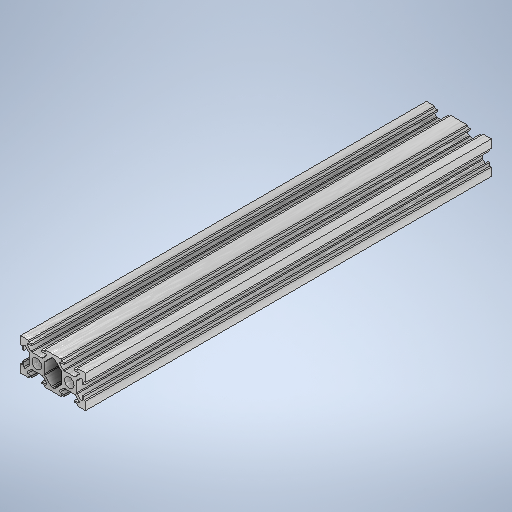
# Autodesk Inventor part: 20x40mm_perfil
Saved by Autodesk Inventor 2025.2 (Build 292293000, 293)
## iProperties
Created: 2025-04-10
Part Number: 20x40mm_perfil
Material: Aço
Document SubType Name: Modeling
Designer: Formação
Density: 7.85 g/cm^3
Appearance: Polido escovado
Author: Formação
Autodesk Inventor part; units mm, degrees
ref_plane "YZ Plane" through (0, 0, 0) normal (1, 0, 0) x (0, 1, 0)
ref_plane "XZ Plane" through (0, 0, 0) normal (0, 1, 0) x (-1, 0, 0)
ref_plane "XY Plane" through (0, 0, 0) normal (0, 0, 1) x (1, 0, 0)
sketch "Esboço1" plane through (0, 0, 0) normal (0, 0, 1) x (1, 0, 0)
  line L0 (1376.0742, -3.2) -> (1376.0729, -2.2)
  line L1 (-14.9742, 1386.056) -> (-13.9742, 1386.056)
  line L2 (-13.9742, 1386.056) -> (-13.9742, 1387.2256)
  line L3 (-13.9742, 1387.2256) -> (-15.9742, 1387.2256)
  line L4 (1376.0625, 5) -> (1376.0625, 4)
  line L5 (1376.0625, 4) -> (2769.8011, 4)
  line L6 (2769.8011, 4) -> (2769.8055, 6)
  arc A0 (-16.3152, 1388.0487) -> (-15.9742, 1387.2256) centre (-15.9742, 1387.7078) ccw
  line L7 (-14.9742, -1386.056) -> (-13.9742, -1386.056)
  line L8 (-13.9742, -1386.056) -> (6.3334, -2779.6467)
  line L9 (6.3334, -2779.6467) -> (4.3336, -2779.6758)
  arc A1 (4.3336, -2779.6758) -> (4.0107, -2780.3971) centre (4.3399, -2780.1116) ccw
  line L10 (4.0107, -2780.3971) -> (5.4731, -2781.7335)
  arc A2 (2770.6738, 6.0529) -> (2769.8055, 6) centre (2770.2413, 5.999) ccw
  line L11 (-20, 10) -> (0, 10) construction
  line L12 (0, 10) -> (0, -10) construction
  line L13 (0, -10) -> (-20, -10) construction
  line L14 (-20, -10) -> (-20, 10) construction
  line L15 (-20, 10) -> (0, -10) construction
  line L16 (0, 10) -> (-20, -10) construction
  line L17 (0, 10) -> (20, 10) construction
  line L18 (20, 10) -> (20, -10) construction
  line L19 (20, -10) -> (0, -10) construction
  line L20 (0, -10) -> (0, 10) construction
  line L21 (0, 10) -> (20, -10) construction
  line L22 (20, 10) -> (0, -10) construction
  circle A3 centre (-10, 0) radius 3 construction
  circle A4 centre (10, 0) radius 3 construction
  line L23 (-20, 10) -> (-20, 5)
  line L24 (-20, -10) -> (-20, -5)
  line L25 (-20, -5) -> (-19, -5)
  line L26 (-19, -5) -> (-19, -3.1)
  line L27 (-19, -3.1) -> (-18, -3.1)
  line L28 (-20, 5) -> (-19, 5)
  line L29 (-19, 5) -> (-19, 3.1)
  line L30 (-19, 3.1) -> (-18, 3.1)
  line L31 (20, -10) -> (20, -5)
  line L32 (20, -5) -> (19, -5)
  line L33 (19, -5) -> (19, -3.1)
  line L34 (19, -3.1) -> (18, -3.1)
  line L35 (20, 10) -> (20, 5)
  line L36 (20, 5) -> (19, 5)
  line L37 (19, 5) -> (19, 3.1)
  line L38 (19, 3.1) -> (18, 3.1)
  line L39 (-18, 3.1) -> (-18, 5.6)
  line L40 (-18, -3.1) -> (-18, -5.6)
  line L41 (18, -3.1) -> (18, -5.6)
  line L42 (18, 3.1) -> (18, 5.6)
  arc A5 (18, 5.6) -> (17.0646, 5.9536) centre (17.4655, 5.6) ccw
  line L43 (-20, -10) -> (-15, -10)
  line L44 (-20, 10) -> (-15, 10)
  line L45 (-15, 10) -> (-15, 9)
  line L46 (-15, 9) -> (-13.1, 9)
  line L47 (-13.1, 9) -> (-13.1, 8)
  line L48 (-13.1, 8) -> (-15.6, 8)
  line L49 (-15, -10) -> (-15, -9)
  line L50 (-15, -9) -> (-13.1, -9)
  line L51 (-13.1, -9) -> (-13.1, -8)
  line L52 (-13.1, -8) -> (-15.6, -8)
  line L53 (-20, 0) -> (20, 0) construction
  line L54 (20, -10) -> (15, -10)
  line L55 (15, -10) -> (15, -9)
  line L56 (15, -9) -> (13.1, -9)
  line L57 (13.1, -9) -> (13.1, -8)
  line L58 (13.1, -8) -> (15.6, -8)
  line L59 (20, 10) -> (15, 10)
  arc A6 (-17.1464, 5.9536) -> (-18, 5.6) centre (-17.5, 5.6) ccw
  arc A7 (-15.9536, -7.1464) -> (-15.6, -8) centre (-15.6, -7.5) ccw
  arc A8 (15.6, -8) -> (15.9536, -7.1464) centre (15.6, -7.5) ccw
  arc A9 (-13.1, -4.6243) -> (-13.6657, -4.8586) centre (-13.1, -5.4243) ccw
  line L60 (-15.9536, -7.1464) -> (-13.6657, -4.8586)
  arc A10 (-18, -5.6) -> (-17.1465, -5.9536) centre (-17.5, -5.6) ccw
  line L61 (-14.6243, 3.1) -> (-14.6243, -3.1) construction
  arc A11 (-14.8586, -3.6657) -> (-14.6243, -3.1) centre (-15.4243, -3.1) ccw
  line L62 (-17.1465, -5.9536) -> (-14.8586, -3.6657)
  arc A12 (-15.6, 8) -> (-15.9536, 7.1464) centre (-15.6, 7.5) ccw
  line L63 (-14.6243, 3.1) -> (-14.6243, -3.1)
  arc A13 (-14.6243, 3.1) -> (-14.8586, 3.6657) centre (-15.4243, 3.1) ccw
  line L64 (-17.1464, 5.9536) -> (-14.8586, 3.6657)
  line L65 (-14.8586, 3.6657) -> (-14.8586, 3.6657)
  arc A14 (-13.6657, 4.8586) -> (-13.1, 4.6243) centre (-13.1, 5.4243) ccw
  line L66 (-15.9536, 7.1464) -> (-13.6657, 4.8586)
  line L67 (-6.9, -9) -> (-6.9, -8)
  line L68 (-6.9, -8) -> (-4.4, -8)
  line L69 (-6.9, -9) -> (-5, -9)
  line L70 (-5, -9) -> (-5, -10)
  line L71 (-10, 0) -> (-10, -10) construction
  arc A15 (-4.4, -8) -> (-4.0464, -7.1464) centre (-4.4, -7.5) ccw
  line L72 (-4.0464, -7.1464) -> (-6.3343, -4.8586)
  arc A16 (-6.3343, -4.8586) -> (-6.9, -4.6243) centre (-6.9, -5.4243) ccw
  line L73 (-13.1, -4.6243) -> (-6.9, -4.6243)
  line L74 (-13.1, 4.6243) -> (-6.9, 4.6243)
  arc A17 (-6.9, 4.6243) -> (-6.3343, 4.8586) centre (-6.9, 5.4243) ccw
  line L75 (-6.3343, 4.8586) -> (-4.0464, 7.1464)
  arc A18 (-4.0464, 7.1464) -> (-4.4, 8) centre (-4.4, 7.5) ccw
  line L76 (-4.4, 8) -> (-6.9, 8)
  line L77 (-6.9, 8) -> (-6.9, 9)
  line L78 (-6.9, 9) -> (-5, 9)
  line L79 (-5, 9) -> (-5, 10)
  line L80 (15, 10) -> (15, 9)
  line L81 (15, 9) -> (13.1, 9)
  line L82 (13.1, 9) -> (13.1, 8)
  line L83 (13.1, 8) -> (15.6, 8)
  arc A19 (15.9536, 7.1464) -> (15.6, 8) centre (15.6, 7.5) ccw
  arc A20 (17.1464, -5.9536) -> (18, -5.6) centre (17.5, -5.6) ccw
  line L84 (13.6657, -4.8586) -> (15.9536, -7.1464)
  line L85 (17.1464, -5.9536) -> (14.8586, -3.6657)
  arc A21 (14.6247, -3.0725) -> (14.8586, -3.6657) centre (15.4243, -3.1) ccw
  arc A22 (13.6657, -4.8586) -> (13.1, -4.6243) centre (13.1, -5.4243) ccw
  line L86 (15.9536, 7.1464) -> (13.6657, 4.8586)
  arc A23 (13.1, 4.6243) -> (13.6657, 4.8586) centre (13.1, 5.4243) ccw
  line L87 (17.0646, 5.9536) -> (14.7767, 3.6657)
  arc A24 (14.7767, 3.6657) -> (14.6247, 3.0725) centre (15.4167, 3.1857) ccw
  line L88 (14.6247, 3.0725) -> (14.6247, -3.0725)
  line L89 (13.1, -4.6243) -> (6.8983, -4.6243)
  arc A25 (6.8983, -4.6243) -> (6.3326, -4.8586) centre (6.8983, -5.4243) ccw
  line L90 (6.3326, -4.8586) -> (4.0448, -7.1464)
  arc A26 (4.0448, -7.1464) -> (4.3983, -8) centre (4.3983, -7.5) ccw
  line L91 (13.1, 4.6243) -> (6.8983, 4.6243)
  arc A27 (6.3326, 4.8586) -> (6.8983, 4.6243) centre (6.8983, 5.4243) ccw
  line L92 (6.3326, 4.8586) -> (4.0448, 7.1464)
  arc A28 (4.3983, 8) -> (4.0448, 7.1464) centre (4.3983, 7.5) ccw
  line L93 (4.3983, 8) -> (6.8983, 8)
  line L94 (4.3983, -8) -> (6.8983, -8)
  line L95 (6.8983, 8) -> (6.8983, 9)
  line L96 (6.8983, 9) -> (4.9983, 9)
  line L97 (4.9983, 9) -> (4.9983, 10)
  line L98 (-5, 10) -> (4.9983, 10)
  line L99 (6.8983, -8) -> (6.8983, -9)
  line L100 (6.8983, -9) -> (5, -9)
  line L101 (5, -9) -> (5, -10)
  line L102 (-5, -10) -> (5, -10)
  line L103 (-5.3777, 3.1) -> (-5.3777, -3.1)
  arc A29 (-5.1434, 3.6657) -> (-5.3777, 3.1) centre (-4.5777, 3.1) ccw
  line L104 (-5.1434, 3.6657) -> (-1.1176, 7.6913)
  arc A30 (-0.3722, 8) -> (-1.1176, 7.6913) centre (-0.3723, 6.9459) ccw
  line L105 (-0.3722, 8) -> (0.3723, 8)
  arc A31 (-5.3777, -3.1) -> (-5.1434, -3.6657) centre (-4.5777, -3.1) ccw
  line L106 (-5.1434, -3.6657) -> (-1.1176, -7.6913)
  arc A32 (-1.1176, -7.6913) -> (-0.3723, -8) centre (-0.3723, -6.9459) ccw
  line L107 (-0.3723, -8) -> (0.3723, -8)
  arc A33 (0.3723, -8) -> (1.1176, -7.6913) centre (0.3723, -6.9459) ccw
  line L108 (1.1176, -7.6913) -> (5.1434, -3.6657)
  arc A34 (5.1434, -3.6657) -> (5.3777, -3.1) centre (4.5777, -3.1) ccw
  line L109 (5.3777, -3.1) -> (5.3777, 3.1)
  arc A35 (5.3777, 3.1) -> (5.1435, 3.6656) centre (4.5777, 3.1) ccw
  line L110 (5.1435, 3.6656) -> (1.1178, 7.6913)
  arc A36 (1.1178, 7.6913) -> (0.3723, 8) centre (0.3725, 6.946) ccw
  circle A37 centre (-10, 0) radius 3
  circle A38 centre (10, 0) radius 3
  point P0 (2769.8033, 5)
  point P1 (2072.9318, 4)
  point P2 (-16.4197, 1387.5232)
  point P3 (0, 0)
  point P4 (0, 0)
  point P5 (-10, 0)
  point P6 (10, 0)
  point P7 (0, 0)
  point P8 (0, 0)
  point P9 (-18.5, 3.1)
  point P10 (-18.5, -3.1)
  point P11 (-19.5, 5)
  point P12 (-19.5, -5)
  point P13 (-19, -4.05)
  point P14 (-19, 4.05)
  point P15 (18.5, -3.1)
  point P16 (19.5, 5)
  point P17 (19.5, -5)
  point P18 (18.5, 3.1)
  point P19 (19, 4.05)
  point P20 (19, -4.05)
  point P21 (17.6545, 6.1)
  point P22 (14.35, -8)
  point P23 (-14.35, -8)
  point P24 (-18, -4.35)
  point P25 (18, -4.35)
  point P26 (-14.6243, 0)
  point P27 (-13.4061, 4.6852)
  point P28 (0, 10)
  point P29 (-10, -10)
  point P30 (-6.9, -8.5)
  point P31 (-13.1, -8.5)
  point P32 (-5.1904, 6.0025)
  point P33 (-14.8096, 6.0025)
  point P34 (-5.1904, -6.0025)
  point P35 (-14.8096, -6.0025)
  point P36 (-10, 4.6243)
  point P37 (-10, -4.6243)
  point P38 (-5.65, 8)
  point P39 (-14.35, 8)
  point P40 (-5, 9.5)
  point P41 (-5, -9.5)
  point P42 (13.1, 8.5)
  point P43 (13.1, -8.5)
  point P44 (14.05, 9)
  point P45 (-5.95, 9)
  point P46 (14.35, 8)
  point P47 (14.8096, -6.0025)
  point P48 (16.0619, 7.6913)
  point P49 (14.8096, 6.0025)
  point P50 (13.4061, -4.6852)
  point P51 (17.9665, 6.0025)
  point P52 (5.1887, -6.0025)
  point P53 (6.5922, 4.6852)
  point P54 (6.5922, -4.6852)
  point P55 (14.6247, 0)
  point P56 (-14.6243, 0)
  point P57 (5.1887, 6.0025)
  point P58 (3.9364, 7.6913)
  point P59 (-3.9381, 7.6913)
  point P60 (5.6483, -8)
  point P61 (5.6483, 8)
  point P62 (5.9483, 9)
  point P63 (5, -9.5)
  point P64 (-5.3777, 0)
  point P65 (-0.7756, 7.9198)
  point P66 (-3.1305, 5.6785)
  point P67 (-3.1305, -5.6785)
  point P68 (0, -8)
  point P69 (0, 0)
  point P70 (0.7756, -7.9198)
  point P71 (-0.7756, -7.9198)
  point P72 (-4.0464, -7.1464)
  point P73 (4.3983, 8)
  dimension "d27" = 135
  dimension "d74" = 2
  dimension "d75" = 1
  dimension "d90" = 20
  dimension "d93" = 20
  dimension "d94" = 40
  dimension "d95" = 20
  dimension "d96" = 6
  dimension "d98" = 6
  dimension "d104" = 5
  dimension "d107" = 6.2
  dimension "d108" = 5
  dimension "d110" = 1
  dimension "d114" = 2.5
  dimension "d115" = 2.5
  dimension "d116" = 1
  dimension "d119" = 0.5
  dimension "d120" = 5
  dimension "d121" = 5
  dimension "d122" = 1.9
  dimension "d123" = 1
  dimension "d124" = 2.5
  dimension "d125" = 1.9
  dimension "d126" = 2.5
  dimension "d127" = 5
  dimension "d128" = 2.5
  dimension "d129" = 1.9
  dimension "d132" = 1
  dimension "d133" = 1
  dimension "d134" = 0.5
  dimension "d135" = 135
  dimension "d136" = 0.5
  dimension "d137" = 1
  dimension "d138" = 1
  dimension "d139" = 135
  dimension "d140" = 0.5
  dimension "d141" = 135
  dimension "d143" = 0.8
  dimension "d144" = 45
  dimension "d145" = 0.5
  dimension "d153" = 45
  dimension "d155" = 0.5
  dimension "d156" = 135
  dimension "d158" = 45
  dimension "d163" = 2.5
  dimension "d164" = 1.9
  dimension "d167" = 0.8
  dimension "d169" = 45
  dimension "d172" = 2.5
  dimension "d173" = 1
  dimension "d174" = 0.5
  dimension "d175" = 0.8
  dimension "d179" = 0.8
  dimension "d181" = 0.8
  dimension "d185" = 0.5
  dimension "d186" = 135
  dimension "d187" = 45
  dimension "d188" = 2.5
  dimension "d189" = 2.5
  dimension "d190" = 1.9
  dimension "d192" = 0.8
  dimension "d193" = 45
  dimension "d194" = 45
  dimension "d195" = 0.9738
  constraints: 222 end point, 82 point on circle, 61 midpoint, 42 horizontal alignment, 42 tangent, 39 centre point, 30 perpendicular, 25 equal length, 21 horizontal, 20 vertical alignment, 16 vertical, 13 equal radius, 13 point on line, 12 coincident, 8 parallel, 1 collinear, 13 other
  measures "d74" distance of L2.end L3.end
  measures "d75" distance of L4.start L4.end
  measures "d90" distance of L12.end L13.end
  measures "d93" distance of L17.end L18.end
  measures "d94" distance of L17.end L11.start
  measures "d95" distance of L13.end L11.start
  measures "d96" diameter of A3
  measures "d98" diameter of A4
  measures "d104" distance of L18.end L31.end
  measures "d107" distance of L27.end L30.end
  measures "d108" distance of L17.end L35.end
  measures "d110" horizontal distance of L32.end L35.end
  measures "d114" distance of L34.end L41.end
  measures "d115" distance of L38.end L42.end
  measures "d116" distance of L38.end L37.end
  measures "d119" vertical distance of point (17.654, 6.1) A5.centre
  measures "d120" distance of L13.end L43.end
  measures "d121" distance of L11.start L44.end
  measures "d122" distance of L45.end L46.end
  measures "d123" distance of L46.end L47.end
  measures "d124" distance of L47.end L48.end
  measures "d125" distance of L49.end L50.end
  measures "d126" distance of L51.end L52.end
  measures "d127" distance of L18.end L54.end
  measures "d128" distance of L57.end L58.end
  measures "d129" distance of L55.end L56.end
  measures "d132" distance of L25.end L24.end
  measures "d133" distance of L27.end L26.end
  measures "d134" radius of A6
  measures "d136" radius of A7
  measures "d137" distance of L56.end L57.end
  measures "d138" distance of L54.end L55.end
  measures "d140" radius of A8
  measures "d143" radius of A9
  measures "d145" radius of A10
  measures "d155" radius of A12
  measures "d163" distance of L67.end L68.end
  measures "d164" distance of L67.start L69.end
  measures "d167" radius of A16
  measures "d172" distance of L76.start L76.end
  measures "d173" distance of L76.end L77.end
  measures "d174" radius of A20
  measures "d175" radius of A21
  measures "d179" radius of A23
  measures "d181" radius of A24
  measures "d185" radius of A26
  measures "d188" distance of L93.start L93.end
  measures "d189" distance of L94.start L94.end
  measures "d190" distance of L95.end L96.end
  measures "d192" radius of A29
  measures "d195" vertical distance of point (-0.776, 7.92) A30.centre
extrude "Extrusão1" add sketch "Esboço1" along normal mid plane 250
